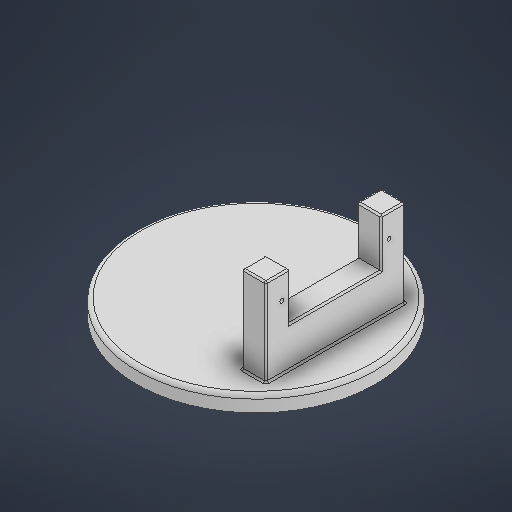
# Autodesk Inventor part: Shoulder
Saved by Autodesk Inventor 2026 (Build 300175000, 175)
## iProperties
Created: 2026-02-13
Part Number: Shoulder
Material: Generisch
Document SubType Name: Modeling
Designer: Jakob Dorninger
Density: 1 g/cm^3
Appearance: Vorgabe
Author: Jakob Dorninger
Autodesk Inventor part; units mm, degrees
ref_plane "YZ Plane" through (0, 0, 0) normal (1, 0, 0) x (0, 1, 0)
ref_plane "XZ Plane" through (0, 0, 0) normal (0, 1, 0) x (-1, 0, 0)
ref_plane "XY Plane" through (0, 0, 0) normal (0, 0, 1) x (1, 0, 0)
sketch "Skizze1" plane through (0, 0, 0) normal (0, 0, 1) x (1, 0, 0)
  circle A0 centre (0, 0) radius 30
  dimension "d0" = 60
  constraints: 1 centre point, 1 coincident
  measures "d0" diameter of A0
extrude "Extrusion1" add sketch "Skizze1" along normal blind 4
sketch "Skizze2" plane through (0, 0, 4) normal (0, 0, 1) x (1, 0, 0)
  line L0 (14, 17.5) -> (20, 17.5)
  line L1 (20, -17.5) -> (14, -17.5)
  line L2 (20, 11.5) -> (14, 11.5)
  line L3 (20, -11.5) -> (14, -11.5)
  line L4 (-42, 0) -> (42, 0) projected
  line L5 (14, -17.5) -> (14, -11.5)
  line L6 (14, 11.5) -> (14, 17.5)
  line L7 (20, 17.5) -> (20, 11.5)
  line L8 (20, -11.5) -> (20, -17.5)
  point P0 (0, 0)
  point P1 (14, 0)
  dimension "d5" = 6
  dimension "d6" = 35
  dimension "d9" = 23
  dimension "d10" = 14
  constraints: 16 end point, 5 parallel, 4 perpendicular, 2 horizontal, 2 vertical alignment, 1 horizontal alignment, 1 point on line, 2 other
  measures "d5" distance of L0.start L0.end
  measures "d6" distance of L0.end L1.start
  measures "d9" distance between parallel lines of L3 L2
  measures "d10" distance from line of point (0, 0) L6
extrude "Extrusion2" add sketch "Skizze2" along normal blind 22
sketch "Skizze3" plane through (14, -17.5, 4) normal (-1, 0, 0) x (0, 0, 1)
  line L0 (22, 35) -> (22, 29) projected
  line L1 (22, 6) -> (22, 0) projected
  line L2 (0, 0) -> (22, 0) projected
  line L3 (-4, 17.5) -> (14.084, 17.5)
  line L4 (0, -12.5) -> (0, 47.5) projected
  point P0 (16, 4)
  point P1 (16, 31)
  point P2 (22, 3)
  point P3 (22, 32)
  dimension "d13" = 27
  dimension "d14" = 16
  constraints: 2 end point, 2 midpoint, 1 horizontal, 1 symmetric about line, 1 vertical alignment
  measures "d13" distance of point (16, 4) point (16, 31)
  measures "d14" distance from line of L4 point (16, 31)
hole "Bohrung1" at (14, -13.5, 20) at (14, 13.5, 20) direction (1, 0, 0) diameter 1 depth 6.5 tip angle 118
fillet "Rundung2" radius 1 1 edges at (-30, 0, 4)
sketch "Skizze6" plane through (14, 11.5, 4) normal (-1, 0, 0) x (0, 0, 1)
  line L0 (0, -23) -> (22, -23) projected
  line L1 (0, 0) -> (22, 0) projected
  line L2 (0, 0) -> (10, 0)
  line L3 (10, 0) -> (10, -23)
  line L4 (10, -23) -> (0, -23)
  line L5 (0, -23) -> (0, 0)
  point P0 (-4, -11.5)
  point P1 (0.5, -23)
  point P2 (21.5, -23)
  point P3 (21.5, 0)
  point P4 (0.5, -23)
  point P5 (10, 0)
  dimension "d30" = 10
  constraints: 8 end point, 2 parallel, 1 horizontal, 1 perpendicular, 1 point on line
  measures "d30" distance of L3.end L0.start
extrude "Extrusion4" add sketch "Skizze6" against normal up to surface (6 mm away)
chamfer "Fasen2" distance 0.4 angle 45 8 edges at (14, 11.5, 20) (17, 11.5, 26) (20, 11.5, 20) (14, 0, 14) (14, -11.5, 20) (17, -11.5, 26) (20, -11.5, 20) (20, 0, 14)
fillet "Rundung3" radius 0.4 14 edges at (14, 0, 4) (14, -17.5, 15) (20, -17.5, 15) (17, -17.5, 26) (20, -14.7, 26) (14, -14.7, 26) (14, 14.7, 26) (20, 14.7, 26) (17, 17.5, 26) (14, 17.5, 15) (17, -17.5, 4) (20, 17.5, 15) (20, 0, 4) (17, 17.5, 4)
